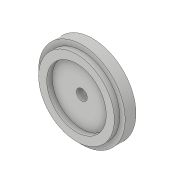
# Autodesk Inventor part: 2sides
Saved by Autodesk Inventor 2022 Beta2 (Build 260130000, 130) ContinuousBuild 0
## iProperties
Created: 2016-02-04
Part Number: 2sides
Material: Generic
Document SubType Name: Modeling
Designer: jmacmillan
Density: 1 g/cm^3
Appearance: Default
Author: jmacmillan
Autodesk Inventor part; units mm, degrees
ref_plane "YZ Plane" through (0, 0, 0) normal (1, 0, 0) x (0, 1, 0)
ref_plane "XZ Plane" through (0, 0, 0) normal (0, 1, 0) x (-1, 0, 0)
ref_plane "XY Plane" through (0, 0, 0) normal (0, 0, 1) x (1, 0, 0)
sketch "Sketch1" plane through (0, 0, 0) normal (0, 0, 1) x (1, 0, 0)
  circle A0 centre (0, 0) radius 25.4
  dimension "d0" = 50.8
  constraints: 1 centre point, 1 coincident
  measures "d0" diameter of A0
extrude "Extrusion1" add sketch "Sketch1" along normal blind 6.35
sketch "Sketch2" plane through (0, 0, 6.35) normal (0, 0, 1) x (1, 0, 0)
  circle A0 centre (0, 0) radius 17.4625
  circle A1 centre (0, 0) radius 22.225
  dimension "d3" = 34.925
  dimension "d4" = 44.45
  constraints: 2 centre point, 2 coincident
  measures "d3" diameter of A0
  measures "d4" diameter of A1
extrude "Extrusion2" add sketch "Sketch2" along normal blind 3.175
sketch "Sketch3" plane through (0, 0, 0) normal (0, 0, -1) x (-1, 0, 0)
  line L0 (-15.875, 0) -> (-7.9375, 13.7482)
  line L1 (-7.9375, 13.7482) -> (7.9375, 13.7482)
  line L2 (7.9375, 13.7482) -> (15.875, 0)
  line L3 (15.875, 0) -> (7.9375, -13.7482)
  line L4 (7.9375, -13.7482) -> (-7.9375, -13.7482)
  line L5 (-7.9375, -13.7482) -> (-15.875, 0)
  circle A0 centre (0, 0) radius 6.35
  line L6 (0, -35.56) -> (0, 35.56) projected
  line L7 (-35.56, 0) -> (35.56, 0) projected
  dimension "d7" = 15.875
  dimension "d8" = 12.7
  constraints: 12 end point, 2 coincident, 1 centre point, 1 horizontal, 1 symmetric about line, 12 other
  measures "d7" distance of L3.end L4.end
  measures "d8" diameter of A0
extrude "Extrusion3" add sketch "Sketch3" along normal blind 6.35 contours L7 A0 L6 L4 L5 | L0 L1 L6 A0 L7 | L1 L2 L7 A0 L6 | L6 A0 L7 L3 L4
hole "Hole1" at (0, 0, 6.35) direction (0, 0, -1) diameter 6.35 end through all
body "Solid1"
